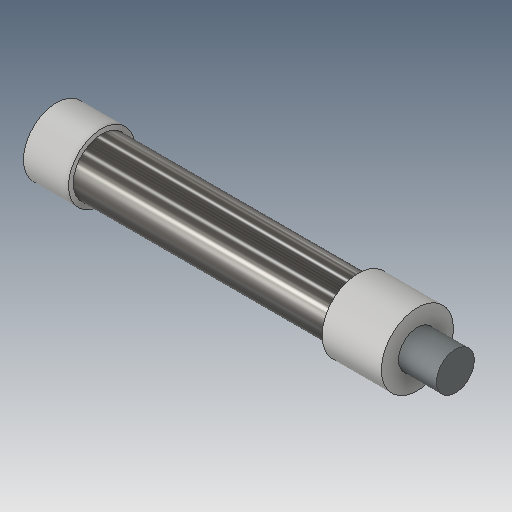
# Autodesk Inventor part: 30mmCylinder
Saved by Autodesk Inventor 2017 (Build 210142000, 142)
## iProperties
Created: 2018-05-01
Part Number: 30mmCylinder
Material: Generic
Document SubType Name: Modeling
Designer: Luiz Gustavo
Density: 1 g/cm^3
Appearance: Default
Mass: 9.95355 g
Surface Area: 39.1624 cm^2
Volume: 9.95355 cm^3
parA: 15,000 mm
parB: 12,000 mm
parC: 14,000 mm
parD: 4,000 mm
parF: 8,000 mm
parGA: 8,000 mm
parGB: 5,000 mm
parH: 28,000 mm
parMM: 4,000 mm
parNA: 12,500 mm
parNB: 9,500 mm
Ndh8: 8,000 mm
parNN: 8,000 mm
parS: 46,000 mm
parZ: 74,000 mm
stroke: 30,000 mm
Author: Luiz Gustavo
Autodesk Inventor part; units mm, degrees
ref_plane "YZ Plane" through (0, 0, 0) normal (1, 0, 0) x (0, 1, 0)
ref_plane "XZ Plane" through (0, 0, 0) normal (0, 1, 0) x (-1, 0, 0)
ref_plane "XY Plane" through (0, 0, 0) normal (0, 0, 1) x (1, 0, 0)
sketch "Sketch1" plane through (0, 0, 0) normal (0, 1, 0) x (-1, 0, 0)
  line L0 (-38, 0) -> (38, 0)
  line L1 (38, 0) -> (38, 7)
  line L2 (38, 7) -> (28.5, 7)
  line L3 (28.5, 7) -> (28.5, 6)
  line L4 (28.5, 6) -> (-25.5, 6)
  line L5 (-38, 7.5926) -> (-38, 0)
  line L6 (-25.5, 6) -> (-25.5, 7.5926)
  line L7 (-25.5, 7.5926) -> (-38, 7.5926)
  point P0 (0, 0)
  point P1 (0, 0)
  dimension "d0" = 76
  dimension "d1" = 9.5
  dimension "d3" = 12.5
  dimension "d4" = 14
  dimension "d5" = 12
  constraints: 16 end point, 3 perpendicular, 3 vertical, 2 horizontal, 1 coincident, 1 midpoint
  measures "d0" distance of L0.start L0.end
  measures "d1" distance of L1.end L2.end
  measures "d3" distance of L6.end L5.start
  measures "d4" diameter of L2 L0
  measures "d5" diameter of L4 L0
revolve "Revolution1" add sketch "Sketch1" angle 360 about axis through (38, 0, 0) along (-1, 0, 0)
sketch "Sketch2" plane through (0, 0, 0) normal (0, 1, 0) x (-1, 0, 0)
  line L0 (-38, -7.5926) -> (-38, 7.5926) projected
  line L1 (38, -7) -> (38, 7) projected
  line L2 (-38, 0) -> (38, 0) construction
  circle A0 centre (-30, 0) radius 2.5
  circle A1 centre (33, 0) radius 2.5
  point P0 (0, 0)
  dimension "d7" = 8
  dimension "d8" = 5
  dimension "d9" = 5
  dimension "d10" = 5
  constraints: 2 centre point, 2 end point, 2 midpoint, 2 point on line
  measures "d7" distance from line of L0 A0.centre
  measures "d8" distance from line of L1 A1.centre
  measures "d9" diameter of A0
  measures "d10" diameter of A1
extrude "Extrusion1" cut sketch "Sketch2" against normal through all
sketch "Sketch3" plane through (38, 0, 0) normal (1, 0, 0) x (0, 0, -1)
  circle A0 centre (0, 0) radius 4
  dimension "d13" = 8
  constraints: 1 centre point, 1 coincident
  measures "d13" diameter of A0
extrude "Extrusion2" add sketch "Sketch3" along normal blind 8
equation "\"d0\" = parS + stroke"
equation "\"d1\" = parNB"
equation "\"d3\" = parNA"
equation "\"d4\" = parC"
equation "\"d5\" = parB"
equation "\"d7\" = parGA"
equation "\"d8\" = parGB"
equation "\"parA\" = 15"
equation "\"parB\" = 12"
equation "\"parC\" = 14"
equation "\"parD\" = 4"
equation "\"parF\" = 8"
equation "\"parGA\" = 8"
equation "\"parGB\" = 5"
equation "\"parH\" = 28"
equation "\"parMM\" = 4"
equation "\"parNA\" = 12.5"
equation "\"parNB\" = 9.5"
equation "\"Ndh8\" = 8"
equation "\"parNN\" = 8"
equation "\"parS\" = 46"
equation "\"parZ\" = 74"
equation "\"stroke\" = 30"
body "Solid1"
